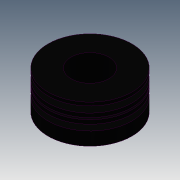
# Autodesk Inventor part: 321527B00000G
Saved by Autodesk Inventor 2015 SP1 (Build 190203100, 203)
## iProperties
Created: 2015-06-04
Material: ALUMINUM, 6061-T651
Vendor: AAVID THERMALLOY
Document SubType Name: Modeling
Designer: ARNOLDJ
Density: 2.7 g/cm^3
Appearance: Anodized - Black
Description: HEAT SINK FOR TO-5 / TO-39 LED
Part Number: 321527B00000G
Project: COMMON
RuleStatus: InUse
AfterDocSave0: file://Part Number Cleaner
LAB/DEPT: COMMON
REQUESTING SCIENTIST: COMMON
SURFACE ROUGHNESS: N/A
DESIGN DEPARTMENT: HHMI: JRC - ID&F
SPECIAL FINISH: NONE
ALTERED ITEM PART NUMBER: N/A
ALTERED ITEM VENDOR: N/A
ALTERED ITEM DESCRIPTION: N/A
Author: ARNOLDJ
Revision Number: 0
Autodesk Inventor part; units mm, degrees
ref_plane "YZ Plane" through (0, 0, 0) normal (1, 0, 0) x (0, 1, 0)
ref_plane "XZ Plane" through (0, 0, 0) normal (0, 1, 0) x (-1, 0, 0)
ref_plane "XY Plane" through (0, 0, 0) normal (0, 0, 1) x (1, 0, 0)
sketch "Sketch1" plane through (0, 0, 0) normal (0, 0, 1) x (1, 0, 0)
  line L0 (0, 0) -> (0, 9.4488)
  line L1 (3.7846, 0) -> (3.7846, 1.27)
  line L2 (3.7846, 0) -> (9.525, 0)
  line L3 (9.525, 0) -> (9.525, 2.9972)
  line L4 (9.525, 2.9972) -> (6.2332, 2.9972)
  line L5 (6.2332, 2.9972) -> (6.2332, 4.3307)
  line L6 (6.2332, 4.3307) -> (9.525, 4.3307)
  line L7 (9.525, 4.3307) -> (9.525, 5.2197)
  line L8 (9.525, 5.2197) -> (5.1664, 5.2197)
  line L9 (4.8819, 1.27) -> (3.7846, 1.27)
  line L10 (5.1664, 5.2197) -> (5.1664, 5.6388)
  line L11 (5.1664, 5.6388) -> (9.525, 5.6388)
  line L12 (9.525, 5.6388) -> (9.525, 6.5278)
  line L13 (9.525, 6.5278) -> (6.2332, 6.5278)
  line L14 (6.2332, 6.5278) -> (6.2332, 7.9248)
  line L15 (6.2332, 7.9248) -> (9.525, 7.9248)
  line L16 (9.525, 7.9248) -> (9.525, 8.6868)
  line L17 (9.525, 8.6868) -> (4.2799, 8.6868)
  line L18 (4.2799, 8.6868) -> (4.2799, 1.778)
  line L19 (4.8819, 1.778) -> (4.8819, 1.27)
  line L20 (4.2799, 1.778) -> (4.8819, 1.778)
  dimension "d0" = 19.05
  dimension "d1" = 7.5692
  dimension "d2" = 1.27
  dimension "d3" = 0
  dimension "d4" = 8.5598
  dimension "d5" = 0.508
  dimension "d6" = 2.9972
  dimension "d7" = 1.3335
  dimension "d8" = 0.889
  dimension "d9" = 0.762
  dimension "d10" = 0.889
  dimension "d11" = 1.397
  dimension "d12" = 8.6868
  constraints: 42 end point, 14 perpendicular, 4 point on line, 4 vertical, 2 vertical alignment, 1 horizontal
  measures "d0" diameter of L3 L0
  measures "d1" diameter of L1 L0
  measures "d2" distance of L1.start L1.end
  measures "d3" distance from line of L0.start L2
  measures "d4" diameter of L18 L0
  measures "d5" distance between parallel lines of L20 L9
  measures "d6" distance of L2.end L3.end
  measures "d7" distance of L4.end L5.end
  measures "d8" distance of L6.end L7.end
  measures "d9" distance of L15.end L16.end
  measures "d10" distance of L11.end L12.end
  measures "d11" distance of L13.end L14.end
  measures "d12" distance between parallel lines of L2 L17
revolve "Revolution1" add sketch "Sketch1" angle 360 about axis through (0, 0, 0) along (0, 1, 0)
sketch "Sketch2" plane through (0, 0, 0) normal (0, 1, 0) x (-1, 0, 0)
  circle A0 centre (0, 0) radius 7.9375 construction
  point P0 (-7.9375, 0)
  point P1 (7.9375, 0)
  dimension "d14" = 15.875
  constraints: 2 point on circle, 1 centre point, 1 coincident
  measures "d14" diameter of A0
hole "Hole1" at (7.9375, 0, 0) at (-7.9375, 0, 0) direction (0, 1, 0) diameter 1.7018 depth 2.54 tip angle 118
body "Solid1"
